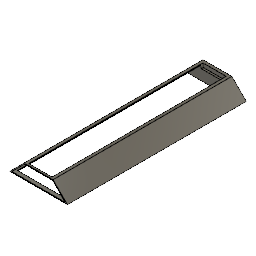
nerf based hopper housing V2 v9 (Autodesk Fusion 360 design; units mm, degrees)
Autodesk Fusion 360 part; units mm, degrees
sketch "top hopper side" plane through (0, 0, 0) normal (0, 1, 0) x (1, 0, 0)
  line L0 (-76.2, 0) -> (0, 0)
  line L1 (0, 0) -> (-19.05, -19.05)
  line L2 (-19.05, -19.05) -> (-57.15, -19.05)
  line L3 (-57.15, -19.05) -> (-76.2, 0)
  dimension "d12" = 76.2
  dimension "d13" = 38.1
  dimension "d14" = 45
  constraint horizontal L0
  constraint parallel L0 L2
  constraint perpendicular L1 L3
  constraint coincident L0.end L1.start
  measures "d12" distance of L0.start L0.end
  measures "d13" distance of L1.end L2.end
  measures "d14" angle of L0 L1
extrude "Extrude3" add sketch "top hopper side" along normal blind 234.95
sketch "side cutout" plane through (0, 0, 0) normal (0, -1, 0) x (1, 0, 0)
  line L0 (-19.05, 19.05) -> (-57.15, 19.05)
  line L1 (-57.15, 19.05) -> (-76.2, 0)
  line L2 (-76.2, 0) -> (0, 0)
  line L3 (0, 0) -> (-19.05, 19.05)
  line L4 (-76.2, 0) -> (-57.15, 19.05)
  line L5 (-19.05, 19.05) -> (0, 0)
  line L6 (-76.2, 0) -> (0, 0)
  line L7 (-57.15, 19.05) -> (-19.05, 19.05)
  line L8 (-73.1339, 1.27) -> (-3.0661, 1.27)
  line L9 (-19.5761, 17.78) -> (-3.0661, 1.27)
  line L10 (-56.6239, 17.78) -> (-19.5761, 17.78)
  line L11 (-73.1339, 1.27) -> (-56.6239, 17.78)
  dimension "d17" = 1.27
  constraint coincident L1.end L2.start
  constraint coincident L0.end L1.start
  constraint coincident L0.start L3.end
  constraint coincident L2.end L3.start
extrude "Extrude4" cut sketch "side cutout" against normal blind 228.6 contours L8 L9 L10 L11
sketch "bottom cutout" plane through (0, 0, 0) normal (0, 0, -1) x (1, 0, 0)
  line L0 (0, 0) -> (-76.2, 0)
  line L1 (-76.2, 0) -> (-76.2, -234.95)
  line L2 (-76.2, -234.95) -> (0, -234.95)
  line L3 (0, -234.95) -> (0, 0)
  line L4 (-5.08, -5.08) -> (-70.7474, -5.08)
  line L5 (-70.7474, -5.08) -> (-70.7474, -228.6)
  line L6 (-5.08, -228.6) -> (-5.08, -5.08)
  line L7 (-5.08, -228.6) -> (-70.7474, -228.6)
  dimension "d20" = 223.52
  dimension "d21" = 65.6674
  dimension "d22" = 5.08
  dimension "d23" = 5.08
  constraint horizontal L4
  constraint vertical L5
  constraint vertical L6
  constraint perpendicular L5 L7
  measures "d20" distance of L4.start L6.start
  measures "d21" distance of L5.end L6.start
  measures "d22" distance of L3 L6
  measures "d23" distance of L0 L4
extrude "Extrude5" cut sketch "bottom cutout" against normal blind 2.54 contours L4 L5 L6 L7
sketch "top cutout" plane through (0, 0, 19.05) normal (0, 0, 1) x (-1, 0, 0)
  line L0 (57.15, 0) -> (19.05, 0)
  line L1 (19.05, 0) -> (19.05, -234.95)
  line L2 (19.05, -234.95) -> (57.15, -234.95)
  line L3 (57.15, -234.95) -> (57.15, 0)
  line L4 (53.34, -2.54) -> (22.86, -2.54)
  line L5 (22.86, -2.54) -> (22.86, -231.14)
  line L6 (22.86, -231.14) -> (53.34, -231.14)
  line L7 (53.34, -231.14) -> (53.34, -2.54)
  dimension "d26" = 228.6
  dimension "d27" = 30.48
  dimension "d28" = 3.81
  dimension "d29" = 2.54
  constraint horizontal L4
  constraint vertical L5
  constraint horizontal L6
  constraint vertical L7
  measures "d26" distance of L4.start L6.end
  measures "d27" distance of L5.end L6.end
  measures "d28" distance of L3 L7
  measures "d29" distance of L0 L4
extrude "Extrude6" cut sketch "top cutout" against normal blind 5.08 contours L4 L5 L6 L7
named bodies: "top hopper"
